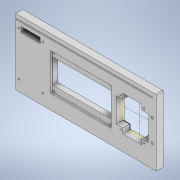
# Autodesk Inventor part: 2020-02-23 CubeBaseFront
Saved by Autodesk Inventor 2020 (Build 240168000, 168)
## iProperties
Created: 2019-12-01
Part Number: 2020-02-23 CubeBaseFront
Material: Generic
Document SubType Name: Modeling
Designer: torto
Density: 1 g/cm^3
Appearance: Default
length: 228.600 mm
height: 107.950 mm
d3: 6.350 mm
d4: 6.350 mm
d5: 222.250 mm
d6: 1.524 mm
spacing: 35.983 mm
d9: 6.350 mm
d10: 3.500 mm
d11: 2.000 ul
d13: 35.983 mm
thickness: 12.700 mm
d19: 0.00 deg
d21: 6.350 mm
d22: 6.350 mm
d23: 222.250 mm
d24: 1.524 mm
d25: 6.350 mm
d26: 0.00 deg
d33: 6.350 mm
d34: 35.983 mm
ScrewDiameter: 4.000 mm
d36: 6.350 mm
d37: 35.983 mm
d38: 3.500 mm
d39: 12.700 mm
d40: 0.00 deg
d49: 105.924 mm
d50: 53.975 mm
LcdLength: 97.409 mm
LcdHeight: 39.878 mm
LcdBorderHeight: 60.325 mm
LcdBorderLength: 98.425 mm
d66: 9.900 mm
d67: 0.00 deg
LcdPcbThickness: 2.800 mm
d69: 0.00 deg
LcdFrameHoleOffset: 2.500 mm
d71: 2.500 mm
LcdFrameHoleDiameter: 3.000 mm
LcdScrewDepth: 6.000 mm
d74: 0.00 deg
InputHeight: 57.150 mm
InputLength: 52.324 mm
InputThickness: 1.600 mm
d78: 0.00 deg
InputHoleSpacing: 0.172 in
d80: 0.278 in
InputScrewDiameter: 3.500 mm
d82: 14.100 mm
d83: 8.500 mm
d84: 11.100 mm
d85: 0.00 deg
InputHoleSpacingX: 7.050 mm
InputHoleSpacingY: 4.250 mm
ScrewDiameterUntapped: 3.500 mm
ScrewCapDiameter: 3.500 mm
PcbThickness: 1.651 mm
TopScrewDiameter: 4.000 mm
InputScrewDiameterUntapped: 2.500 mm
InputScrewDiameterFull: 3.500 mm
InputCornerLengthX: 10.700 mm
InputCornerLengthY: 8.500 mm
Author: torto
Autodesk Inventor part; units mm, degrees
ref_plane "YZ Plane" through (0, 0, 0) normal (1, 0, 0) x (0, 1, 0)
ref_plane "XZ Plane" through (0, 0, 0) normal (0, 1, 0) x (-1, 0, 0)
ref_plane "XY Plane" through (0, 0, 0) normal (0, 0, 1) x (1, 0, 0)
sketch "Sketch1" plane through (0, 0, 0) normal (0, 0, 1) x (1, 0, 0)
  line L0 (0, 0) -> (228.6, 0)
  line L1 (228.6, 0) -> (228.6, 107.95)
  line L2 (228.6, 107.95) -> (0, 107.95)
  line L3 (0, 107.95) -> (0, 0)
  line L4 (228.6, 107.95) -> (222.25, 107.95) construction
  line L5 (222.25, 107.95) -> (222.25, 101.6) construction
  line L6 (222.25, 101.6) -> (228.6, 101.6) construction
  line L7 (228.6, 101.6) -> (228.6, 107.95) construction
  line L8 (222.25, 101.6) -> (0, 101.6)
  line L9 (0, 101.6) -> (0, 100.076)
  line L10 (0, 100.076) -> (222.25, 100.076)
  line L11 (222.25, 100.076) -> (222.25, 101.6)
  line L12 (228.6, 0) -> (222.25, 0) construction
  line L13 (222.25, 0) -> (222.25, 35.9833) construction
  line L14 (222.25, 35.9833) -> (228.6, 35.9833) construction
  line L15 (228.6, 35.9833) -> (228.6, 0) construction
  circle A0 centre (222.25, 35.9833) radius 2
  circle A1 centre (222.25, 71.9667) radius 2
  dimension "length" = 228.6
  dimension "height" = 107.95
  dimension "d3" = 6.35
  dimension "d4" = 6.35
  dimension "d5" = 222.25
  dimension "d6" = 1.524
  dimension "spacing" = 35.9833
  dimension "d9" = 6.35
  dimension "TopScrewDiameter" = 4
  dimension "d13" = 35.9833
  constraints: 32 end point, 8 parallel, 4 horizontal, 4 perpendicular, 2 centre point, 2 coincident, 1 vertical, 3 other
  measures "length" distance of L2.end L1.end
  measures "height" distance of L1.end L0.end
  measures "d3" distance of L5.end L4.end
  measures "d4" distance of L5.end L6.end
  measures "d5" distance of L10.end L9.end
  measures "d6" distance of L9.end L8.end
  measures "spacing" distance of L12.end L13.end
  measures "d9" distance of L13.end L14.end
  measures "TopScrewDiameter" diameter of A0
  measures "d13" distance of A0.centre A1.centre
extrude "Generic Shape" add sketch "Sketch1" along normal blind 12.7
chamfer "Chamfer Outside Edges" distance 1.5 angle 45 3 edges at (114.3, 107.95, 0) (228.6, 107.95, 6.35) (228.6, 53.975, 0)
sketch "ScrewCapDiameter" plane through (0, 0, 0) normal (0, 0, -1) x (-1, 0, 0)
  circle A0 centre (-222.25, 71.9667) radius 2 projected
  circle A1 centre (-222.25, 71.9667) radius 3.5
  circle A2 centre (-222.25, 35.9833) radius 2 projected
  circle A3 centre (-222.25, 35.9833) radius 3.5
  point P0 (0, 0)
  dimension "d106" = 7
  dimension "d107" = 7
  constraints: 2 centre point, 2 coincident
  measures "d106" diameter of A1
  measures "d107" diameter of A3
extrude "ScrewCapCountersink" cut sketch "ScrewCapDiameter" against normal blind 4
sketch "PcbNotchDimensions" plane through (0, 0, 12.7) normal (0, 0, 1) x (1, 0, 0)
  line L0 (228.6, 107.95) -> (0, 107.95) construction
  line L1 (228.6, 107.95) -> (222.25, 107.95) construction
  line L2 (222.25, 107.95) -> (222.25, 101.6) construction
  line L3 (222.25, 101.6) -> (228.6, 101.6) construction
  line L4 (228.6, 101.6) -> (228.6, 107.95) construction
  line L5 (222.25, 101.6) -> (0, 101.6)
  line L6 (0, 101.6) -> (0, 99.949)
  line L7 (0, 99.949) -> (222.25, 99.949)
  line L8 (222.25, 99.949) -> (222.25, 101.6)
  point P0 (0, 0)
  dimension "d21" = 6.35
  dimension "d22" = 6.35
  dimension "d23" = 222.25
  dimension "PcbThickness" = 1.651
  constraints: 16 end point, 4 parallel, 2 horizontal, 2 perpendicular
  measures "d21" distance of L2.end L1.end
  measures "d22" distance of L2.end L3.end
  measures "d23" distance of L7.end L6.end
  measures "PcbThickness" distance of L6.end L5.end
extrude "PCB Notch" cut sketch "PcbNotchDimensions" against normal blind 6.35
sketch "UntappedScrewHoleDimensions" plane through (0, 0, 0) normal (-1, 0, 0) x (0, 0, 1)
  line L0 (0, 0) -> (6.35, 0) construction
  line L1 (6.35, 0) -> (6.35, 35.9833) construction
  line L2 (6.35, 35.9833) -> (0, 35.9833) construction
  line L3 (0, 35.9833) -> (0, 0) construction
  circle A0 centre (6.35, 35.9833) radius 1.75
  line L4 (0, 107.95) -> (6.35, 107.95) construction
  line L5 (6.35, 107.95) -> (6.35, 71.9667) construction
  line L6 (6.35, 71.9667) -> (0, 71.9667) construction
  line L7 (0, 71.9667) -> (0, 107.95) construction
  circle A1 centre (6.35, 71.9667) radius 1.75
  dimension "d33" = 6.35
  dimension "d34" = 35.9833
  dimension "ScrewDiameterUntapped" = 3.5
  dimension "d36" = 6.35
  dimension "d37" = 35.9833
  dimension "d38" = 3.5
  constraints: 16 end point, 4 parallel, 2 centre point, 2 coincident, 2 horizontal, 2 perpendicular
  measures "d33" distance of L2.end L1.end
  measures "d34" distance of L1.end L0.end
  measures "ScrewDiameterUntapped" diameter of A0
  measures "d36" distance of L5.end L6.end
  measures "d37" distance of L4.end L5.end
  measures "d38" diameter of A1
extrude "UntappedScrewDepth" cut sketch "UntappedScrewHoleDimensions" against normal blind 12.7
sketch "LCD" plane through (0, 0, 0) normal (0, 0, -1) x (-1, 0, 0)
  line L0 (0, 0) -> (-228.6, 0) construction
  line L1 (0, 0) -> (-105.924, 0) construction
  line L2 (-105.924, 0) -> (-105.924, 53.975) construction
  line L3 (-105.924, 53.975) -> (0, 53.975) construction
  line L4 (0, 53.975) -> (0, 0) construction
  line L5 (-154.6285, 73.914) -> (-57.2195, 73.914)
  line L6 (-57.2195, 73.914) -> (-57.2195, 34.036)
  line L7 (-57.2195, 34.036) -> (-154.6285, 34.036)
  line L8 (-154.6285, 34.036) -> (-154.6285, 73.914)
  line L9 (-154.6285, 73.914) -> (-57.2195, 34.036) construction
  line L10 (-57.2195, 73.914) -> (-154.6285, 34.036) construction
  line L11 (-155.1365, 84.1375) -> (-56.7115, 84.1375)
  line L12 (-56.7115, 84.1375) -> (-56.7115, 23.8125)
  line L13 (-56.7115, 23.8125) -> (-155.1365, 23.8125)
  line L14 (-155.1365, 23.8125) -> (-155.1365, 84.1375)
  line L15 (-155.1365, 84.1375) -> (-56.7115, 23.8125) construction
  line L16 (-56.7115, 84.1375) -> (-155.1365, 23.8125) construction
  dimension "d49" = 105.924
  dimension "d50" = 53.975
  dimension "LcdLength" = 97.409
  dimension "LcdHeight" = 39.878
  dimension "LcdBorderHeight" = 60.325
  dimension "LcdBorderLength" = 98.425
  constraints: 32 end point, 6 parallel, 4 midpoint, 3 horizontal, 3 perpendicular
  measures "d49" distance of L2.end L3.end
  measures "d50" distance of L1.end L2.end
  measures "LcdLength" distance of L6.end L7.end
  measures "LcdHeight" distance of L7.end L5.start
  measures "LcdBorderHeight" distance of L11.end L12.end
  measures "LcdBorderLength" distance of L12.end L13.end
extrude "LcdWindow" cut sketch "LCD" against normal blind 9.9 contours L5 L6 L7 L8
sketch "LcdFrameDimensions" plane through (0, 0, 12.7) normal (0, 0, 1) x (1, 0, 0)
  line L0 (155.1365, 84.1375) -> (56.7115, 84.1375) projected
  line L1 (155.1365, 23.8125) -> (155.1365, 84.1375) projected
  line L2 (56.7115, 23.8125) -> (155.1365, 23.8125) projected
  line L3 (56.7115, 84.1375) -> (56.7115, 23.8125) projected
  point P0 (0, 0)
extrude "LcdFrame" cut sketch "LcdFrameDimensions" against normal blind 2.8
sketch "LcdScrewsSketch" plane through (0, 0, 9.9) normal (0, 0, 1) x (1, 0, 0)
  line L0 (56.7115, 23.8125) -> (56.7115, 84.1375) construction
  line L1 (56.7115, 84.1375) -> (59.2115, 84.1375) construction
  line L2 (59.2115, 84.1375) -> (59.2115, 81.6375) construction
  line L3 (59.2115, 81.6375) -> (56.7115, 81.6375) construction
  line L4 (56.7115, 81.6375) -> (56.7115, 84.1375) construction
  circle A0 centre (59.2115, 81.6375) radius 1.5
  line L5 (56.7115, 84.1375) -> (155.1365, 84.1375) construction
  line L6 (105.924, 84.1375) -> (105.924, 23.8125) construction
  line L7 (155.1365, 23.8125) -> (56.7115, 23.8125) construction
  line L8 (56.7115, 53.975) -> (155.1365, 53.975) construction
  line L9 (155.1365, 84.1375) -> (155.1365, 23.8125) construction
  circle A1 centre (152.6365, 81.6375) radius 1.5
  circle A2 centre (59.2115, 26.3125) radius 1.5
  circle A3 centre (152.6365, 26.3125) radius 1.5
  point P0 (0, 0)
  dimension "LcdFrameHoleOffset" = 2.5
  dimension "d71" = 2.5
  dimension "LcdFrameHoleDiameter" = 3
  constraints: 12 end point, 4 centre point, 4 midpoint, 3 symmetric about line, 2 parallel, 1 coincident, 1 horizontal, 1 perpendicular, 3 other
  measures "LcdFrameHoleOffset" distance of L2.end L3.end
  measures "d71" distance of L1.end L2.end
  measures "LcdFrameHoleDiameter" diameter of A0
extrude "LcdScrews" cut sketch "LcdScrewsSketch" against normal blind 6
sketch "InputDimensions" plane through (0, 0, 0) normal (0, 0, 1) x (1, 0, 0)
  line L0 (154.6285, 34.036) -> (154.6285, 73.914) construction
  line L1 (228.6, 0) -> (228.6, 107.95) construction
  line L2 (163.576, 82.55) -> (215.9, 82.55)
  line L3 (215.9, 82.55) -> (215.9, 25.4)
  line L4 (215.9, 25.4) -> (163.576, 25.4)
  line L5 (163.576, 25.4) -> (163.576, 82.55)
  line L6 (228.6, 107.95) -> (189.738, 107.95) construction
  line L7 (228.6, 53.975) -> (228.6, 107.95) construction
  line L8 (215.9, 82.55) -> (163.576, 25.4) construction
  line L9 (215.9, 25.4) -> (163.576, 82.55) construction
  line L10 (189.738, 53.975) -> (228.6, 53.975) construction
  line L11 (228.6, 53.975) -> (228.6, 107.95) construction
  line L12 (228.6, 107.95) -> (189.738, 107.95) construction
  line L13 (189.738, 107.95) -> (189.738, 53.975) construction
  point P0 (0, 0)
  dimension "InputHeight" = 57.15
  dimension "InputLength" = 52.324
  dimension "d93" = 38.862
  dimension "d94" = 53.975
  constraints: 24 end point, 4 parallel, 3 horizontal, 2 perpendicular, 1 midpoint
  measures "InputHeight" distance of L4.end L2.start
  measures "InputLength" distance of L3.end L4.end
  measures "d93" distance of L10.start L10.end
  measures "d94" distance of L12.end L10.start
extrude "InputCountersink" cut sketch "InputDimensions" along normal blind 1.6
sketch "InputCorners" plane through (0, 0, 1.6) normal (0, 0, -1) x (-1, 0, 0)
  line L0 (-215.9, 25.4) -> (-215.9, 82.55) projected
  line L1 (-215.9, 82.55) -> (-208.85, 82.55) construction
  line L2 (-208.85, 82.55) -> (-208.85, 78.3) construction
  line L3 (-208.85, 78.3) -> (-215.9, 78.3) construction
  line L4 (-215.9, 78.3) -> (-215.9, 82.55) construction
  circle A0 centre (-208.85, 78.3) radius 1.75
  line L5 (-215.9, 82.55) -> (-163.576, 82.55) projected
  line L6 (-189.738, 82.55) -> (-189.738, 25.4) construction
  line L7 (-163.576, 25.4) -> (-215.9, 25.4) projected
  line L8 (-215.9, 53.975) -> (-163.576, 53.975) construction
  line L9 (-163.576, 82.55) -> (-163.576, 25.4) projected
  line L10 (-215.9, 82.55) -> (-205.2, 82.55) construction
  line L11 (-205.2, 82.55) -> (-205.2, 74.05)
  line L12 (-205.2, 74.05) -> (-215.9, 74.05)
  line L13 (-215.9, 74.05) -> (-215.9, 82.55) construction
  line L14 (-174.276, 82.55) -> (-174.276, 74.05)
  line L15 (-174.276, 74.05) -> (-163.576, 74.05)
  line L16 (-205.2, 25.4) -> (-205.2, 33.9)
  line L17 (-205.2, 33.9) -> (-215.9, 33.9)
  line L18 (-174.276, 33.9) -> (-163.576, 33.9)
  line L19 (-174.276, 25.4) -> (-174.276, 33.9)
  circle A1 centre (-208.85, 78.3) radius 1.25
  circle A2 centre (-208.85, 29.65) radius 1.25
  circle A3 centre (-170.626, 78.3) radius 1.25
  circle A4 centre (-170.626, 29.65) radius 1.25
  point P0 (0, 0)
  point P1 (-163.576, 33.9)
  point P2 (-163.576, 74.05)
  point P3 (-215.9, 74.05)
  point P4 (-205.2, 25.4)
  dimension "InputHoleSpacingX" = 7.05
  dimension "InputHoleSpacingY" = 4.25
  dimension "InputScrewDiameterFull" = 3.5
  dimension "InputCornerLengthX" = 10.7
  dimension "InputCornerLengthY" = 8.5
  dimension "InputScrewDiameterUntapped" = 2.5
  constraints: 32 end point, 12 symmetric about line, 5 centre point, 4 midpoint, 4 parallel, 2 coincident, 2 horizontal, 2 perpendicular, 3 other
  measures "InputHoleSpacingX" distance of L2.end L3.end
  measures "InputHoleSpacingY" distance of L1.end L2.end
  measures "InputScrewDiameterFull" diameter of A0
  measures "InputCornerLengthX" distance of L11.end L12.end
  measures "InputCornerLengthY" distance of L10.end L11.end
  measures "InputScrewDiameterUntapped" diameter of A1
extrude "InputCut" cut sketch "InputCorners" against normal blind 11.1 contours L0 L12 L11 L5 L14 L15 L9 L18 L19 L7 L16 L17 | A1 | A2 | A3 | A4
chamfer "LcdChamfer" distance 1.651 angle 45 4 edges at (105.924, 73.914, 0) (154.6285, 53.975, 0) (105.924, 34.036, 0) (57.2195, 53.975, 0)
sketch "KeypadDimensions" plane through (0, 0, 0) normal (0, 0, -1) x (-1, 0, 0)
  line L0 (-48, 94.025) -> (0, 94.025)
  line L1 (0, 94.025) -> (0, 13.925)
  line L2 (0, 13.925) -> (-48, 13.925)
  line L3 (-48, 13.925) -> (-48, 94.025)
  line L4 (-48, 94.025) -> (0, 13.925) construction
  line L5 (-48, 13.925) -> (0, 94.025) construction
  line L6 (0, 99.949) -> (0, 0) construction
  line L7 (0, 0) -> (-24, 0) construction
  line L8 (-24, 0) -> (-24, 53.975) construction
  line L9 (-24, 53.975) -> (0, 53.975) construction
  line L10 (0, 53.975) -> (0, 0) construction
  dimension "KeypadLength" = 48
  dimension "KeypadHeight" = 80.1
  dimension "d97" = 53.975
  dimension "d98" = 24
  constraints: 20 end point, 4 parallel, 2 horizontal, 2 perpendicular, 1 midpoint
  measures "KeypadLength" distance of L0.start L0.end
  measures "KeypadHeight" distance of L2.end L0.start
  measures "d97" distance of L7.end L8.end
  measures "d98" distance of L8.end L9.end
extrude "KeypadCountersink" cut sketch "KeypadDimensions" against normal blind 1.6
sketch "KeypadCorners" plane through (0, 0, 1.6) normal (0, 0, -1) x (-1, 0, 0)
  line L0 (-48, 13.925) -> (-48, 94.025) construction
  line L1 (-48, 94.025) -> (-44.2, 94.025) construction
  line L2 (-44.2, 94.025) -> (-44.2, 89.925) construction
  line L3 (-44.2, 89.925) -> (-48, 89.925) construction
  line L4 (-48, 89.925) -> (-48, 94.025) construction
  circle A0 centre (-44.2, 89.925) radius 1.75 construction
  circle A1 centre (-44.2, 89.925) radius 1.25
  line L5 (-48, 94.025) -> (-39.5, 94.025)
  line L6 (-39.5, 94.025) -> (-39.5, 85.525)
  line L7 (-39.5, 85.525) -> (-48, 85.525)
  line L8 (-48, 85.525) -> (-48, 94.025)
  line L9 (-48, 94.025) -> (0, 94.025) construction
  line L10 (-24, 94.025) -> (-24, 13.925) construction
  line L11 (0, 13.925) -> (-48, 13.925) construction
  line L12 (-48, 53.975) -> (0, 53.975) construction
  line L13 (0, 99.949) -> (0, 0) construction
  line L14 (-8.5, 94.025) -> (-8.5, 85.525)
  line L15 (-8.5, 85.525) -> (0, 85.525)
  line L16 (-39.5, 13.925) -> (-39.5, 22.425)
  line L17 (-39.5, 22.425) -> (-48, 22.425)
  line L18 (-8.5, 22.425) -> (0, 22.425)
  line L19 (-8.5, 13.925) -> (-8.5, 22.425)
  line L20 (-39.5, 85.525) -> (-8.5, 85.525)
  line L21 (0, 94.025) -> (-4.8, 94.025) construction
  line L22 (-4.8, 94.025) -> (-4.8, 89.925) construction
  line L23 (-4.8, 89.925) -> (0, 89.925) construction
  line L24 (0, 89.925) -> (0, 94.025) construction
  line L25 (0, 13.925) -> (-4.8, 13.925) construction
  line L26 (-4.8, 13.925) -> (-4.8, 17.725) construction
  line L27 (-4.8, 17.725) -> (0, 17.725) construction
  line L28 (0, 17.725) -> (0, 13.925) construction
  circle A2 centre (-4.8, 17.725) radius 1.25
  line L29 (-48, 13.925) -> (-44.2, 13.925) construction
  line L30 (-44.2, 13.925) -> (-44.2, 17.725) construction
  line L31 (-44.2, 17.725) -> (-48, 17.725) construction
  line L32 (-48, 17.725) -> (-48, 13.925) construction
  circle A3 centre (-44.2, 17.725) radius 1.25
  circle A4 centre (-4.8, 89.925) radius 1.25
  line L33 (-39.5, 94.025) -> (-8.5, 94.025)
  dimension "LeftKeypadHoleSpacingX" = 3.8
  dimension "UpperKeypadHoleSpacingY" = 4.1
  dimension "KeypadHoleDiameter" = 3.5
  dimension "KeypadScrewHoleDiameterUntapped" = 2.5
  dimension "KeypadCornerLengthX" = 8.5
  dimension "KeypadCornerLengthY" = 8.5
  dimension "RightKeypadHoleSpacingX" = 4.8
  dimension "d118" = 4.1
  dimension "d121" = 4.8
  dimension "LowerKeypadHoleSpacingY" = 3.8
  dimension "d123" = 2.5
  dimension "d124" = 3.8
  dimension "d125" = 3.8
  dimension "d126" = 2.5
  dimension "d127" = 2.5
  constraints: 60 end point, 10 parallel, 9 symmetric about line, 6 horizontal, 6 perpendicular, 5 centre point, 5 coincident, 3 midpoint, 1 collinear, 1 point on line
  measures "LeftKeypadHoleSpacingX" distance of L2.end L3.end
  measures "UpperKeypadHoleSpacingY" distance of L1.end L2.end
  measures "KeypadHoleDiameter" diameter of A0
  measures "KeypadScrewHoleDiameterUntapped" diameter of A1
  measures "KeypadCornerLengthX" distance of L6.end L7.end
  measures "KeypadCornerLengthY" distance of L5.end L6.end
  measures "RightKeypadHoleSpacingX" distance of L23.end L22.end
  measures "d118" distance of L22.end L21.end
  measures "d121" distance of L26.end L27.end
  measures "LowerKeypadHoleSpacingY" distance of L25.end L26.end
  measures "d123" diameter of A2
  measures "d124" distance of L31.end L30.end
  measures "d125" distance of L29.end L30.end
  measures "d126" diameter of A3
  measures "d127" diameter of A4
extrude "Extrusion15" cut sketch "KeypadCorners" against normal blind 11.1 contours A1 | L33 L14 L20 L6 | A2 | A3 | A4
equation "\"d3\" = 0.5 * thickness"
equation "\"d4\" = 0.5 * thickness"
equation "\"d5\" = length - 0.5 * thickness"
equation "\"spacing\" = 0.333333 * height"
equation "\"d9\" = 0.5 * thickness"
equation "\"d13\" = spacing"
equation "\"d25\" = 0.5 * thickness"
equation "\"d33\" = 0.5 * thickness"
equation "\"d34\" = 0.333333 * height"
equation "\"d36\" = 0.5 * thickness"
equation "\"d37\" = 0.333333 * height"
equation "\"d38\" = ScrewDiameterUntapped"
equation "\"d50\" = 0.5 * height"
equation "\"d66\" = thickness - LcdPcbThickness"
equation "\"LcdPcbThickness\" = thickness - LcdThickness"
equation "\"d71\" = LcdFrameHoleOffset"
equation "\"d93\" = thickness + 0.5 * InputLength"
equation "\"d94\" = 0.5 * height"
equation "\"d84\" = thickness - InputThickness"
equation "\"d97\" = 0.5 * height"
equation "\"d98\" = 0.5 * KeypadLength"
equation "\"d99\" = InputThickness"
equation "\"LcdThickness\" = 9.9"
equation "\"thickness\" = 12.7"
equation "\"InputThickness\" = 1.6"
body "Solid1"
